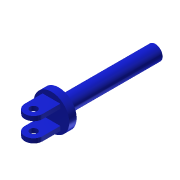
# Autodesk Inventor part: 從動桿
Saved by Autodesk Inventor 2015 SP2 (Build 190223200, 223)
## iProperties
Created: 2020-03-26
Part Number: 從動桿
Material: 一般
Document SubType Name: Modeling
Designer: Kuan-Lun Hsu
Density: 1 g/cm^3
Appearance: 藍色 - 牆面油漆 - 亮面
Mass: 8.45252 g
Surface Area: 43.268 cm^2
Volume: 8.45252 cm^3
Author: Kuan-Lun Hsu
Autodesk Inventor part; units mm, degrees
ref_plane "YZ Plane" through (0, 0, 0) normal (1, 0, 0) x (0, 1, 0)
ref_plane "XZ Plane" through (0, 0, 0) normal (0, 1, 0) x (-1, 0, 0)
sketch "草圖1" plane through (0, 0, 0) normal (0, 0, 1) x (1, 0, 0)
  line L0 (0, 0) -> (5, 0)
  line L1 (5, 0) -> (5, 70)
  line L2 (5, 70) -> (0, 70)
  line L3 (0, 70) -> (0, 0)
  line L4 (0, 0) -> (12, 0)
  line L5 (12, 0) -> (12, 5)
  line L6 (12, 5) -> (0, 5)
  line L7 (0, 5) -> (0, 0)
  dimension "d0" = 10
  dimension "d1" = 70
  dimension "d2" = 5
  dimension "d3" = 12
  constraints: 16 end point, 4 parallel, 2 horizontal, 2 perpendicular
  measures "d0" diameter of L1 L3
  measures "d1" distance of L0.end L1.end
  measures "d2" distance of L4.end L5.end
  measures "d3" distance of L5.end L6.end
revolve "迴轉1" add sketch "草圖1" angle 360 about axis through (0, 70, 0) along (0, -1, 0)
ref_plane "工作平面1" through (0, 0, 5) normal (0, 0, 1) x (1, 0, 0)
sketch "草圖2" plane through (0, 0, 5) normal (0, 0, 1) x (1, 0, 0)
  line L0 (-6, 0) -> (6, 0)
  line L1 (6, 0) -> (6, -12)
  line L2 (6, -12) -> (-6, -12)
  line L3 (-6, -12) -> (-6, 0)
  line L4 (-12, 0) -> (12, 0) projected
  circle A0 centre (0, -12) radius 6
  point P0 (0, 0)
  dimension "d6" = 12
  dimension "d7" = 12
  constraints: 8 end point, 2 midpoint, 2 parallel, 1 horizontal, 1 horizontal alignment, 1 perpendicular, 2 other
  measures "d6" distance of L0.end L1.end
  measures "d7" distance of L1.end L2.end
extrude "擠出1" add sketch "草圖2" along normal blind 3
sketch "草圖3" plane through (0, 0, 8) normal (0, 0, 1) x (1, 0, 0)
  arc A0 (-6, -12) -> (6, -12) centre (0, -12) ccw projected
  circle A1 centre (0, -12) radius 2.5
  point P0 (0, 0)
  dimension "d10" = 5
  constraints: 1 centre point, 1 coincident
  measures "d10" diameter of A1
extrude "擠出2" cut sketch "草圖3" against normal through all
mirror "鏡射1" about plane through (0, 0, 0) normal (0, 0, 1) of "擠出2", "擠出1"
